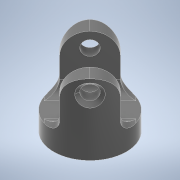
# Autodesk Inventor part: joint
Saved by Autodesk Inventor 2022 (Build 260153000, 153)
## iProperties
Created: 2022-02-15
Part Number: joint
Material: Generic
Document SubType Name: Modeling
Designer: Dahway
Density: 1 g/cm^3
Appearance: Smooth - Black
Author: Dahway
Autodesk Inventor part; units mm, degrees
ref_plane "YZ Plane" through (0, 0, 0) normal (1, 0, 0) x (0, 1, 0)
ref_plane "XZ Plane" through (0, 0, 0) normal (0, 1, 0) x (-1, 0, 0)
ref_plane "XY Plane" through (0, 0, 0) normal (0, 0, 1) x (1, 0, 0)
sketch "Sketch1" plane through (0, 0, 0) normal (0, 1, 0) x (-1, 0, 0)
  circle A0 centre (0, 0) radius 10
  dimension "d0" = 20
  constraints: 1 centre point, 1 coincident
  measures "d0" diameter of A0
extrude "Extrusion1" add sketch "Sketch1" along normal blind 5
sketch "Sketch2" plane through (0, 5, 0) normal (0, 1, 0) x (1, 0, 0)
  circle A0 centre (0, 0) radius 10 projected
  arc A1 (-1.5, 9.8869) -> (-9.8869, 1.5) centre (0, 0) ccw
  line L0 (-9.8869, 1.5) -> (-1.5, 9.8869) construction
  line L1 (-9.8869, 1.5) -> (1.974, 1.5) construction
  line L2 (-9.8869, 1.5) -> (-8.4726, 0.0858)
  line L3 (-9.8869, 1.5) -> (-7.8869, 1.5) construction
  line L4 (-1.5, 9.8869) -> (-0.0858, 8.4726)
  line L5 (-1.5, 9.8869) -> (0.5, 9.8869) construction
  line L6 (-0.0858, 8.4726) -> (-8.4726, 0.0858)
  dimension "d3" = 45
  dimension "d4" = 2
  dimension "d5" = 45
  dimension "d6" = 2
  dimension "d7" = 45
  constraints: 14 end point, 4 point on circle, 3 equal length, 3 horizontal, 2 perpendicular, 1 centre point
  measures "d3" angle of L1 L0
  measures "d4" distance of L0.start L2.end
  measures "d5" angle of L2 L3
  measures "d6" distance of L0.end L4.end
  measures "d7" angle of L4 L5
extrude "Extrusion2" add sketch "Sketch2" along normal blind 14.5 contours L4 L6 L2 A0 picked at (-5.2098, 5.2098)
fillet "Fillet1" radius 3 3 edges at (-0.7929, 5, -9.1798) (-4.2792, 5, -4.2792) (-9.1798, 5, -0.7929)
sketch "Sketch4" plane through (-8.4726, 8, -0.0858) normal (0.7071068, 0, 0.7071068) x (0.7071068, 0, -0.7071068)
  line L0 (0, 11.5) -> (11.8608, 11.5) projected
  line L1 (11.8608, 0) -> (11.8608, 11.5) projected
  point P0 (5.9304, -8)
  point P1 (5.9303, 7.5)
  point P2 (2, 8)
  point P3 (9.8608, 8)
  point P4 (11.8608, 6)
  dimension "d18" = 4
  dimension "d19" = 5.9305
  constraints: 1 other
  measures "d19" distance from line of L1 point (5.93, 7.5)
hole "Hole1" at (-4.2793, 15.5, -4.2791) direction (-0.7071068, 0, -0.7071068) diameter 4 end through all
chamfer "Chamfer1" distance 1 angle 45 1 edges at (-7.5746, 17.3583, -6.5288)
pattern_circular "Circular Pattern2" count 2 over 360 about axis through (0, 0, 0) along (0, 1, 0) of "Extrusion2", "Fillet1", "Hole1", "Chamfer1"
fillet "Fillet5" radius 5.9305 4 edges at (-0.7929, 19.5, -9.1798) (-9.1798, 19.5, -0.7929) (9.1798, 19.5, 0.7929) (0.7929, 19.5, 9.1798)
body "Solid1"
